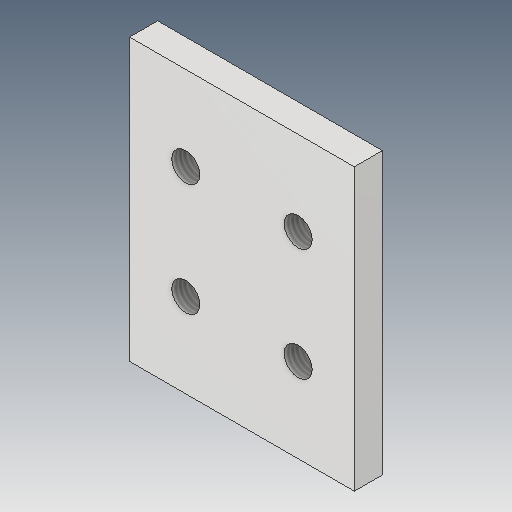
# Autodesk Inventor part: CP010
Saved by Autodesk Inventor 2017 (Build 210142000, 142)
## iProperties
Created: 2017-05-15
Part Number: CP010
Material: ABS Plastic
Document SubType Name: Modeling
Designer: zallen
Density: 1.06 g/cm^3
Appearance: Smooth - White
Mass: 10.1837 g
Surface Area: 50.5708 cm^2
Volume: 9.6073 cm^3
Author: zallen
Autodesk Inventor part; units mm, degrees
ref_plane "YZ Plane" through (0, 0, 0) normal (1, 0, 0) x (0, 1, 0)
ref_plane "XZ Plane" through (0, 0, 0) normal (0, 1, 0) x (-1, 0, 0)
ref_plane "XY Plane" through (0, 0, 0) normal (0, 0, 1) x (1, 0, 0)
sketch "Sketch1" plane through (0, 0, 0) normal (0, 0, 1) x (1, 0, 0)
  line L0 (-20, -25) -> (20, -25)
  line L1 (20, -25) -> (20, 25)
  line L2 (20, 25) -> (-20, 25)
  line L3 (-20, 25) -> (-20, -25)
  line L4 (-20, -25) -> (20, 25) construction
  line L5 (20, -25) -> (-20, 25) construction
  point P0 (0, 0)
  dimension "d0" = 40
  dimension "d1" = 50
  constraints: 12 end point, 2 midpoint, 2 parallel, 1 horizontal, 1 perpendicular
  measures "d0" distance of L2.end L1.end
  measures "d1" distance of L1.end L0.end
extrude "Extrusion1" add sketch "Sketch1" along normal blind 5
sketch "Sketch2" plane through (0, 0, 5) normal (0, 0, 1) x (1, 0, 0)
  circle A0 centre (-10, 10) radius 2.5
  circle A1 centre (-10, -10) radius 2.5
  circle A2 centre (10, 10) radius 2.5
  circle A3 centre (10, -10) radius 2.5
  point P0 (0, 0)
  dimension "d4" = 5
  dimension "d5" = 5
  dimension "d6" = 5
  dimension "d7" = 5
  dimension "d8" = 10
  dimension "d9" = 10
  dimension "d10" = 10
  dimension "d11" = 10
  constraints: 4 centre point, 2 horizontal alignment, 2 vertical alignment
  measures "d4" diameter of A0
  measures "d5" diameter of A1
  measures "d6" diameter of A2
  measures "d7" diameter of A3
  measures "d8" horizontal distance of point (0, 0) A0.centre
  measures "d9" horizontal distance of point (0, 0) A1.centre
  measures "d10" horizontal distance of point (0, 0) A0.centre
  measures "d11" horizontal distance of point (0, 0) A2.centre
extrude "Extrusion2" cut sketch "Sketch2" against normal through all
thread "Thread1" size "M5x0.8" class "6H" standard "ANSI Metric M Profile" full length
thread "Thread2" size "M5x0.8" class "6H" standard "ANSI Metric M Profile" full length
thread "Thread3" size "M5x0.8" class "6H" standard "ANSI Metric M Profile" full length
thread "Thread4" size "M5x0.8" class "6H" standard "ANSI Metric M Profile" full length
body "Solid1"
